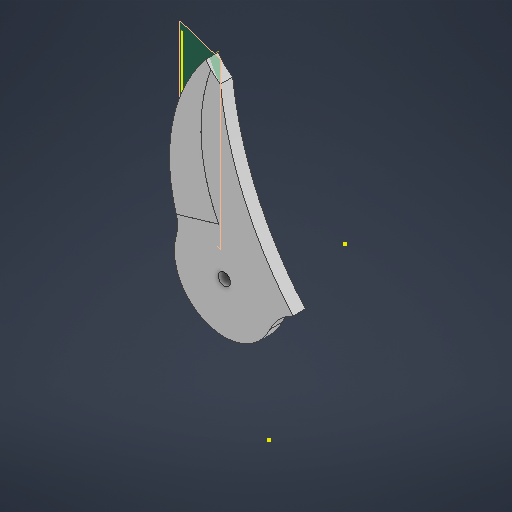
# Autodesk Inventor part: Hoja de Corte
Saved by Autodesk Inventor 2026.1 (Build 301233020, 233B)
## iProperties
Created: 2025-11-03
Part Number: Hoja de Corte
Material: Generic
Document SubType Name: Modeling
Designer: Marcelo
Density: 1 g/cm^3
Appearance: Default
Author: Marcelo
Autodesk Inventor part; units mm, degrees
ref_plane "YZ Plane" through (0, 0, 0) normal (1, 0, 0) x (0, 1, 0)
ref_plane "XZ Plane" through (0, 0, 0) normal (0, 1, 0) x (-1, 0, 0)
ref_plane "XY Plane" through (0, 0, 0) normal (0, 0, 1) x (1, 0, 0)
sketch "Sketch1" plane through (0, 0, 0) normal (0, 0, 1) x (1, 0, 0)
  arc A0 (-12.4355, 76.1693) -> (-19.7198, 39.6098) centre (18.623, 50.9756) ccw
  arc A1 (-12.4355, 76.1693) -> (-8.9, 72.6338) centre (-2.5891, 82.4801) ccw
  line L0 (-12.4355, 76.1693) -> (-8.9, 72.6338) construction
  line L1 (-12.4355, 76.1693) -> (-7.4355, 76.1693) construction
  arc A2 (-8.9, 72.6338) -> (8.9173, 32.3025) centre (65.5817, 81.4365) ccw
  arc A3 (8.9173, 32.3025) -> (3.2604, 26.6457) centre (13.5829, 21.98) ccw
  line L2 (8.9173, 32.3025) -> (3.2604, 26.6457) construction
  line L3 (8.9173, 32.3025) -> (16.9173, 32.3025) construction
  arc A4 (-19.7055, 35.1113) -> (3.2604, 26.6457) centre (-7.92, 31.6991) ccw
  arc A5 (-19.7055, 35.1113) -> (-19.7198, 39.6098) centre (-27.3899, 37.3361) ccw
  circle A6 centre (-7.92, 31.6991) radius 1.5
  line L4 (-21.3689, 76.1693) -> (8.9173, 76.1693)
  line L5 (8.9173, 76.1693) -> (8.9173, 19.4296)
  line L6 (8.9173, 19.4296) -> (-21.3689, 19.4296)
  line L7 (-21.3689, 19.4296) -> (-21.3689, 76.1693)
  line L8 (-21.3689, 39.6098) -> (3.328, 39.6098)
  line L9 (-19.7198, 39.6098) -> (3.328, 39.6098) construction
  line L10 (3.328, 39.6098) -> (3.328, 76.1693)
  line L11 (3.328, 39.6098) -> (39.8875, 39.6098) construction
  dimension "d25" = 39.9919
  dimension "d26" = 5
  dimension "d27" = 45
  dimension "d28" = 75
  dimension "d29" = 8
  dimension "d30" = 135
  dimension "d31" = 8
  dimension "d32" = 3
  dimension "d51" = 0
  dimension "d52" = 90
  constraints: 24 end point, 13 point on circle, 7 centre point, 5 horizontal, 5 point on line, 5 tangent, 3 equal length, 2 parallel, 1 coincident, 1 perpendicular
  measures "d25" radius of A0
  measures "d26" distance of L0.start L0.end
  measures "d27" angle of L0 L1
  measures "d28" radius of A2
  measures "d29" distance of L2.start L2.end
  measures "d30" angle of L2 L3
  measures "d31" radius of A5
  measures "d32" diameter of A6
  measures "d51" distance between parallel lines of L8 L9
  measures "d52" angle of L11 L10
extrude "Extrusion1" add sketch "Sketch1" along normal blind 3 contours A1 A2 L8 A0 | L8 A2 A3 A4 A5
sketch "Sketch2" plane through (0, 0, 0) normal (0, 0, -1) x (-1, 0, 0)
  arc A0 (8.9, 72.6338) -> (12.4355, 76.1693) centre (2.5891, 82.4801) ccw projected
  arc A1 (19.7198, 39.6098) -> (12.4355, 76.1693) centre (-18.623, 50.9756) ccw projected
  arc A2 (-8.9173, 32.3025) -> (8.9, 72.6338) centre (-65.5817, 81.4365) ccw projected
  arc A3 (19.7198, 39.6098) -> (19.7055, 35.1113) centre (27.3899, 37.3361) ccw projected
  line L0 (19.7198, 39.6098) -> (0.1925, 45.3982)
  arc A4 (11.2162, 74.5839) -> (12.4355, 76.1693) centre (2.5891, 82.4801) ccw
  arc A5 (9.3275, 42.6903) -> (11.2162, 74.5839) centre (-26.3268, 60.8045) ccw
  point P0 (0, 0)
  dimension "d35" = 0
  dimension "d37" = 2
  constraints: 6 point on circle, 2 centre point, 2 end point, 2 equal radius, 1 point on line
  measures "d35" distance from line of A1.centre L0
  measures "d37" distance of A0.end A4.start
extrude "Extrusion2" add sketch "Sketch2" along normal blind 0.01 and the other way blind 3.01 contours A0 A1 L0 A5
sketch "Sketch5" plane through (0, 0, 3) normal (0, 0, 1) x (1, 0, 0)
  line L0 (-9.3275, 42.6903) -> (-19.7198, 39.6098) projected
  line L1 (-9.3275, 42.6903) -> (-9.3275, 72.9213)
  arc A0 (-11.2162, 74.5839) -> (-8.9, 72.6338) centre (-2.5891, 82.4801) ccw projected
  line L2 (-9.3275, 42.6903) -> (20.9035, 42.6903) construction
  line L3 (-19.7198, 39.6098) -> (-9.3275, 39.6098)
  line L4 (-19.7198, 39.6098) -> (-9.3275, 39.6098) construction
  line L5 (-9.3275, 39.6098) -> (-9.3275, 42.6903)
  line L6 (-21.3689, 76.1693) -> (-21.3689, 42.6903)
  arc A1 (-12.4355, 76.1693) -> (-19.7198, 39.6098) centre (18.623, 50.9756) ccw projected
  line L7 (-19.7198, 39.6098) -> (-21.3689, 39.6098)
  line L8 (-21.3689, 39.6098) -> (-21.3689, 43.2681)
  line L9 (-21.3689, 76.1693) -> (-9.3275, 76.1693)
  line L10 (-9.3275, 72.9213) -> (-9.3275, 76.1693)
  point P0 (0, 0)
  point P1 (-21.3689, 50.9756)
  dimension "d47" = 90
  dimension "d48" = 0
  constraints: 20 end point, 5 point on line, 3 horizontal, 2 equal length, 2 point on circle, 2 vertical, 1 perpendicular, 1 tangent
  measures "d47" angle of L2 L1
  measures "d48" distance between parallel lines of L3 L4
sketch "Sketch6" plane through (0, 0, -0.01) normal (0, 0, -1) x (-1, 0, 0)
  line L0 (21.3689, 76.1693) -> (21.3689, 42.6903) projected
  arc A0 (19.7198, 39.6098) -> (12.4355, 76.1693) centre (-18.623, 50.9756) ccw projected
  point P0 (0, 0)
  point P1 (21.3689, 50.9756)
  constraints: 1 point on circle, 1 point on line
ref_plane "Work Plane3" through (-9.3275, 76.1693, 3) normal (0.2425094, 0, -0.9701491) x (0, -1, 0)
extrude "Extrusion3" [suppressed]
body "Solid1"
